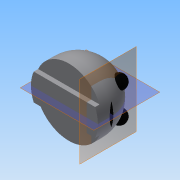
# Autodesk Inventor part: head3
Saved by Autodesk Inventor 2015 (Build 190159000, 159)
## iProperties
Created: 2015-06-18
Part Number: head3
Material: Générique
Document SubType Name: Modeling
Designer: Gregwar
Density: 1 g/cm^3
Appearance: Par défaut
Author: Gregwar
Autodesk Inventor part; units mm, degrees
ref_plane "XZ Plane" through (0, 0, 0) normal (0, 1, 0) x (-1, 0, 0)
ref_plane "XY Plane" through (0, 0, 0) normal (0, 0, 1) x (1, 0, 0)
sketch "Esquisse1" plane through (0, 0, 0) normal (0, 1, 0) x (-1, 0, 0)
  circle A0 centre (0, 0) radius 37.5
  line L0 (37.5, 0) -> (-37.5, 0)
  dimension "d0" = 75
  constraints: 2 end point, 2 point on circle, 1 centre point, 1 coincident, 1 horizontal
  measures "d0" diameter of A0
revolve "Révolution1" add sketch "Esquisse1" angle 180 about axis through (-37.5, 0, 0) along (1, 0, 0) picked at (1.2379, -17.9235) contours A0 L0
sketch "Esquisse3" plane through (0, 0, 0) normal (0, -1, 0) x (1, 0, 0)
  circle A0 centre (0, 0) radius 37.5 projected
extrude "Extrusion2" add sketch "Esquisse3" along normal blind 10
sketch "Esquisse4" plane through (0, -10, 0) normal (0, -1, 0) x (1, 0, 0)
  circle A0 centre (0, 0) radius 37.5 projected
  line L0 (-52.5, 0) -> (52.5, 0) projected
  line L1 (34.3693, 15) -> (-34.3693, 15)
  line L2 (-34.3693, -15) -> (34.3693, -15)
  dimension "d8" = 15
  dimension "d9" = 15
  constraints: 4 end point, 4 point on circle, 2 parallel
  measures "d8" distance between parallel lines of L0 L1
  measures "d9" distance between parallel lines of L0 L2
extrude "Extrusion3" add sketch "Esquisse4" along normal blind 5 contours L0 A0 L1 | A0 L2 L0
ref_plane "Plan de construction1" through (25, 0, 0) normal (1, 0, 0) x (0, 1, 0)
sketch "Esquisse6" plane through (25, 0, 0) normal (1, 0, 0) x (0, 1, 0)
  line L0 (0, 37.5) -> (0, -37.5) projected
  circle A0 centre (21.2908, 16.8449) radius 7.533
  line L1 (27.3087, 12.3138) -> (15.2729, 21.376)
  line L2 (0, 0) -> (47.2705, 0) construction
  constraints: 4 end point, 2 point on circle, 1 centre point, 1 horizontal, 1 midpoint
ref_plane "Plan de construction2" through (34.3693, -10, 0) normal (0, 0, -1) x (-1, 0, 0)
revolve "Révolution2" add sketch "Esquisse6" angle 360 about axis through (25, 27.3087, 12.3138) along (0, -0.7988722, 0.6015008) picked at (22.6507, 18.9558) contours A0 L1
mirror "Symétrie1" about plane through (34.3693, -10, 0) normal (0, 0, -1) of "Révolution2"
sketch "Esquisse8" plane through (25, 0, 0) normal (1, 0, 0) x (0, 1, 0)
  line L0 (-10, -15) -> (-10, -15) construction
  line L1 (-10, -15) -> (-15, -15) construction
  line L2 (-15, 15) -> (-15, -15) construction
  line L3 (-10, 15) -> (-15, 15) construction
  line L4 (-10, 15) -> (-10, 15) construction
  line L5 (-10, 15) -> (-15, 15) construction
  line L6 (-15, -15) -> (-15, 15) construction
  line L7 (-10, -15) -> (-15, -15) construction
  line L8 (0, 37.5) -> (0, -37.5) construction
  line L9 (-15, 15) -> (-15, -15) construction
  line L10 (-15, 0) -> (31.9456, 0) construction
  line L11 (2.3018, 12.6924) -> (2.3018, -12.6924)
  line L12 (2.3018, -12.6924) -> (-5.9689, 0) construction
  line L13 (-5.9689, 0) -> (2.3018, 12.6924) construction
  spline S0 degree 2 poles (2.3018, -12.6924) (-5.9689, 0) (2.3018, 12.6924) knots 1 1 1 2 2 2
  line L14 (2.3018, 0) -> (-5.9689, 0) construction
  point P0 (0, 0)
  constraints: 6 end point, 2 midpoint, 1 coincident, 1 horizontal, 1 perpendicular, 1 point on line, 1 vertical, 3 other
extrude "Extrusion5" cut sketch "Esquisse8" along normal through all
equation "\"d9\" = d8"
